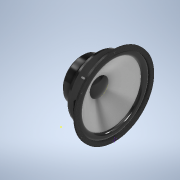
# Autodesk Inventor part: WOOFER
Saved by Autodesk Inventor 2022 (Build 260153000, 153)
## iProperties
Created: 2021-11-01
Part Number: WOOFER
Material: Типовые
Document SubType Name: Modeling
Designer: A
Density: 1 g/cm^3
Appearance: Глянцевая — черная
Author: A
Autodesk Inventor part; units mm, degrees
ref_plane "YZ Plane" through (0, 0, 0) normal (1, 0, 0) x (0, 1, 0)
ref_plane "XZ Plane" through (0, 0, 0) normal (0, 1, 0) x (-1, 0, 0)
ref_plane "XY Plane" through (0, 0, 0) normal (0, 0, 1) x (1, 0, 0)
sketch "Эскиз1" plane through (0, 0, 0) normal (0, 1, 0) x (-1, 0, 0)
  line L0 (83.2087, -239) -> (78.3073, -239)
  line L1 (78.3073, -239) -> (78.3073, -250.4004)
  line L2 (78.3073, -250.4004) -> (83.2087, -250.4004)
  line L3 (83.2087, -250.4004) -> (83.2087, -239)
  line L4 (162.4744, -144.1441) -> (145.5184, -144.1441)
  line L5 (145.5184, -144.1441) -> (145.5184, -198.6323)
  line L6 (145.5184, -198.6323) -> (162.4744, -198.6323)
  line L7 (162.4744, -198.6323) -> (162.4744, -144.1441)
  line L8 (145.5184, -144.1441) -> (138.9918, -144.1441)
  line L9 (138.9918, -144.1441) -> (138.9918, -193.9441)
  line L10 (138.9918, -193.9441) -> (145.5184, -193.9441)
  line L11 (145.5184, -193.9441) -> (145.5184, -144.1441)
  line L12 (167.5745, -144.1441) -> (162.4744, -144.1441)
  line L13 (162.4744, -144.1441) -> (162.4744, -193.9441)
  line L14 (162.4744, -193.9441) -> (167.5745, -193.9441)
  line L15 (167.5745, -193.9441) -> (167.5745, -144.1441)
  line L16 (173.1245, -144.1441) -> (167.5745, -144.1441)
  line L17 (173.1245, -144.1441) -> (167.5745, -144.1441)
  line L18 (167.5745, -144.1441) -> (167.5745, -171.142)
  line L19 (167.5745, -171.142) -> (167.1245, -171.142)
  line L20 (173.1245, -165.142) -> (173.1245, -144.1441)
  arc A0 (167.1245, -171.142) -> (173.1245, -165.142) centre (167.1245, -165.142) ccw
  line L21 (123.8805, -144.1441) -> (119.8729, -144.1441)
  line L22 (173.1245, -144.1441) -> (71.9201, -144.1441)
  line L23 (88, -226) -> (120.1841, -169.2735)
  arc A1 (113.245, -144.1441) -> (120.1841, -169.2735) centre (163.4222, -143.8113) ccw
  line L24 (88, -226) -> (88.7398, -226)
  line L25 (88.7398, -226) -> (120.9239, -169.2735)
  line L26 (138.9918, -186.9213) -> (138.9918, -144.1441)
  line L27 (138.9918, -144.1441) -> (123.8805, -144.1441)
  line L28 (120.1841, -169.2735) -> (138.9918, -169.2735)
  line L29 (138.9918, -169.2735) -> (138.9918, -144.1441)
  line L30 (138.9918, -144.1441) -> (120.1841, -144.1441)
  line L31 (120.1841, -144.1441) -> (120.1841, -169.2735)
  line L32 (120.1841, -169.2735) -> (120.9239, -169.2735)
  line L33 (120.3717, -196) -> (120.1841, -196)
  line L34 (120.1841, -196) -> (125, -196)
  line L35 (125, -196) -> (125, -224)
  line L36 (125, -224) -> (120.1841, -224)
  line L37 (120.1841, -224) -> (120.1841, -196)
  line L38 (120.9239, -169.2735) -> (121.3783, -169.2735)
  line L39 (121.3783, -169.2735) -> (121.3783, -195.8837)
  line L40 (121.3783, -195.8837) -> (120.9239, -195.8837)
  line L41 (120.9239, -195.8837) -> (120.9239, -169.2735)
  arc A2 (88, -226) -> (83.2087, -239) centre (88.4725, -233.5571) ccw
  arc A3 (88.5699, -224.9956) -> (83, -239) centre (88.5553, -233.0996) ccw
  line L42 (83, -239) -> (83.2087, -250.4004)
  point P0 (0, 0)
  point P1 (165.0244, -144.1441)
  point P2 (170.3495, -144.1441)
  point P3 (142.2551, -144.1441)
  point P4 (83.5787, -144.2227)
  point P5 (78.3073, -144.2227)
  point P6 (138.9918, -144.1441)
  point P7 (84.4407, -239.6768)
  point P8 (138.9918, -144.1441)
  point P9 (88.8229, -225)
  point P10 (81.2075, -235.6614)
  dimension "d69" = 49.8
  dimension "d76" = 6.5266
  dimension "d80" = 6
  dimension "d137" = 28
  constraints: 86 end point, 17 parallel, 12 horizontal, 9 point on line, 8 perpendicular, 8 point on circle, 4 centre point, 3 midpoint, 2 tangent, 1 vertical
  measures "d69" distance of L8.end L9.end
  measures "d76" distance of L9.end L10.end
  measures "d80" radius of A0
  measures "d137" distance of L34.end L35.end
revolve "Вращение1" add sketch "Эскиз1" angle 360 about axis through (-173.1245, 0, -144.1441) along (1, 0, 0) contours L3 L42 L0 | L0 A3 L23 A2 | L42 L2 L1 L0 | L23 L28 L25 L24 | L31 L21 L22 L9 L28 | A1 L22 L21 L31 | L28 L39 L40 L41 | L9 L8 L5 L10 | L4 L7 L6 L5 | L12 L15 A0 L19 L14 L7 | L16 L20 A0 L15 | L34 L35 L36 L37 L33
sketch "Эскиз2" plane through (-78.3073, 0, -144.1441) normal (1, 0, 0) x (0, 0, -1)
  line L0 (0.2128, 146.7196) -> (0.2128, -156.6622)
  circle A0 centre (0, 0) radius 68.2205 projected
  point P0 (-144.1441, 0)
  constraints: 2 end point, 1 coincident, 1 vertical
sketch "Эскиз3" plane through (-78.3073, 0, -144.1441) normal (1, 0, 0) x (0, 0, -1)
  point P0 (-144.1441, 0)
  point P1 (0.1683, -101.7218)
hole "Отверстие1" at (-78.3073, -101.7218, -144.3124) direction (-1, 0, 0) diameter 4 end through all counterbore diameter 6 counterbore depth 3
pattern_circular "Круговой массив1" count 6 over 360 about axis through (-88.3699, 0, -144.1441) along (1, 0, 0) of "Вращение1", "Отверстие1"
sketch "Эскиз4" plane through (-78.3073, 0, -144.1441) normal (1, 0, 0) x (0, 0, -1)
  point P0 (-144.1441, 0)
  point P1 (0, -102)
hole "Отверстие2" at (-78.3073, -102, -144.1441) direction (-1, 0, 0) diameter 4 end through all counterbore diameter 6 counterbore depth 3
sketch "Эскиз5" plane through (-81.3073, -102, -144.1441) normal (1, 0, 0) x (0, 0, -1)
  circle A0 centre (0, 102) radius 106.1777 projected
  circle A1 centre (0, 102) radius 106.2563 projected
  point P0 (-144.1441, 102)
sketch "Эскиз6" plane through (0, 0, 0) normal (0, 1, 0) x (-1, 0, 0)
  line L0 (83.5787, -38.0451) -> (83.5787, -250.4004) projected
  line L1 (120.1276, -178.333) -> (120.1276, -212.4432) projected
  line L2 (83.5787, -250.4004) -> (120.1276, -212.4432)
  line L3 (120.1276, -212.4432) -> (120.1276, -199)
  line L4 (120.1276, -198) -> (104, -224)
  line L5 (104, -224) -> (83.5787, -247)
  line L6 (83.5787, -247) -> (83.5787, -250.4004)
  line L7 (120.1276, -198) -> (120.1276, -212.4432)
  line L8 (123.8805, -175.5513) -> (123.8805, -206.8799) projected
  line L9 (138.9918, -169.0441) -> (138.9918, -193.9441) projected
  line L10 (123.8805, -206.8799) -> (138.9918, -193.9441)
  line L11 (138.9918, -193.9441) -> (138.9918, -187)
  line L12 (138.9918, -187) -> (127.9984, -196.4108)
  line L13 (127.9984, -196.4108) -> (123.8805, -196.4108)
  line L14 (123.8805, -196.4108) -> (123.8805, -206.8799)
  point P0 (0, 0)
  constraints: 22 end point, 3 point on line, 2 parallel, 2 perpendicular, 1 collinear
extrude "Выдавливание1" add sketch "Эскиз6" along normal mid plane 4
pattern_circular "Круговой массив2" count 8 over 360 about axis through (-163.4222, 0, -144.1441) along (1, 0, 0) of "Выдавливание1"
